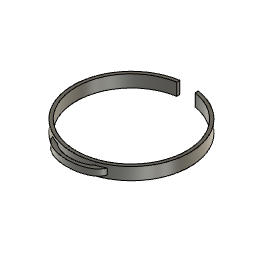
anchor_ring v2 (Autodesk Fusion 360 design; units mm, degrees)
Autodesk Fusion 360 part; units mm, degrees
sketch "Sketch1" plane through (0, 0, 0) normal (0, 0, 1) x (1, 0, 0)
  line L0 (1.5, 8.8741) -> (1.5, 9.3808)
  line L1 (-1.5, 9.3808) -> (-1.5, 8.8741)
  line L2 (-5.476, 0) -> (5.476, 0)
  arc A0 (-1.5, 8.8741) -> (1.5, 8.8741) centre (0, 0) ccw
  arc A1 (-1.5, 9.3808) -> (1.5, 9.3808) centre (0, 0) ccw
  line L3 (0, 7) -> (0, -7)
  dimension "d1" = 18
  dimension "d2" = 19
  dimension "d5" = 3
  constraint coincident A0.centre A1.centre
  constraint vertical L0
  constraint vertical L1
  constraint perpendicular L1 L2
  constraint perpendicular L2 L3
  constraint symmetric L0 L1 L3
  constraint midpoint A0.centre L3
  constraint midpoint A0.centre L2
  measures "d1" diameter of A0
  measures "d2" diameter of A1
  measures "d5" distance of L0 L1
extrude "Extrude1" add sketch "Sketch1" along normal blind 2
sketch "Sketch2" plane through (0, 0, 0) normal (0, 1, 0) x (1, 0, 0)
sketch "Sketch3" plane through (0, 0, 2) normal (0, 0, 1) x (-1, 0, 0)
  line L0 (1.5, -8.8741) -> (1.5, -9.3808)
  arc A0 (1.5, -9.3808) -> (-1.5, -9.3808) centre (0, 0) ccw
  line L1 (-1.5, -9.3808) -> (-1.5, -8.8741)
  arc A1 (1.5, -8.8741) -> (-1.5, -8.8741) centre (0, 0) ccw
  line L2 (7.8349, 0) -> (-7.8349, 0)
  line L3 (0, -10.7948) -> (0, 10.7948)
  line L4 (5, 9.25) -> (-5, 9.25)
  ellipse E0 centre (0, 8) end of major axis (-4.5, 8) minor radius 2.5
  line L5 (4.5, 8) -> (-4.5, 8)
  line L6 (0, 10.5) -> (0, 5.5)
  ellipse E1 centre (0, 8) end of major axis (-3.5, 8) minor radius 2
  line L7 (3.5, 8) -> (-3.5, 8)
  line L8 (0, 10) -> (0, 6)
  dimension "d10" = 10
  dimension "d11" = 18.5
  dimension "d15" = 9
  dimension "d16" = 5
  dimension "d17" = 7
  dimension "d18" = 4
  dimension "d23" = 2.5
  constraint horizontal L2
  constraint vertical L3
  constraint midpoint L2 A0.centre
  constraint midpoint L3 A0.centre
  constraint symmetric L3 L4.start L4.end
  constraint coincident E0 L5.start
  constraint coincident E0 L6.start
  constraint coincident E0 L6.end
  constraint coincident L3 E0.centre
  constraint coincident E1 L7.start
  constraint coincident E1 L7.end
  constraint coincident E1 L8.start
  constraint coincident E1 L8.end
  constraint concentric E0 E1
  measures "d10" distance of L4.start L4.end
  measures "d15" distance of E0
  measures "d17" distance of E1
extrude "Extrude2" add sketch "Sketch3" against normal blind 1 from surface at -0.5 contours A1 L3 E0 L5 L6 E1 | A1 E0 L5 | A0 A1 E0 L5 E1 | A0 L4 E0 E1 | A1 L5 E1 | A1 L3 E0 L5 L6 E1 | A0 A1 L3 L4 L6 E1 L8 | A0 L4 E1 | L3 L4 E0 L6 E1 | A1 L3 L5 L6 E1 L7 L8 | L3 L5 L6 E1 L7 L8 | L3 L5 L6 E1 L7 L8 | A1 E0 L5 | A0 L3 L4 L6 L8 | A0 L3 L4 L6 E1 L8 | L3 L4 E0 L6 E1 | A1 L3 L5 L6 E1 L7 L8 | A0 A1 L3 L4 L6 E1 L8 | A1 L5 E1 | A0 A1 E0 L5 E1 | A0 L3 L4 L6 L8 | A0 L3 L4 L6 E1 L8 | A0 L4 E0 E1 | A0 L4 E1
delete_face "DeleteFace1" 1 faces at (0, -7.8167, 1.5)
extrude "Extrude3" cut sketch "Sketch3" against normal blind 1 from surface at -0.5 contours A0 L4 E1 | A0 L3 L4 L6 E1 L8 | A0 L3 L4 L6 E1 L8 | A0 L4 E1
